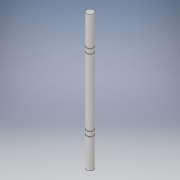
# Autodesk Inventor part: Förderbandwelle_hinten
Saved by Autodesk Inventor 2018 (Build 220112000, 112)
## iProperties
Created: 2017-12-01
Part Number: Förderbandwelle_hinten
Material: Generisch
Document SubType Name: Modeling
Designer: Dominik
Density: 1 g/cm^3
Appearance: Vorgabe
Author: Dominik
Autodesk Inventor part; units mm, degrees
ref_plane "YZ Plane" through (0, 0, 0) normal (1, 0, 0) x (0, 1, 0)
ref_plane "XY Plane" through (0, 0, 0) normal (0, 0, 1) x (1, 0, 0)
sketch "Skizze1" plane through (0, 0, 0) normal (0, 0, 1) x (1, 0, 0)
  circle A0 centre (0, 0) radius 5
  dimension "d0" = 10
  constraints: 1 centre point, 1 coincident
  measures "d0" diameter of A0
extrude "Extrusion1" add sketch "Skizze1" along normal blind 100
sketch "Skizze4" plane through (0, 0, 0) normal (0, 0, -1) x (-1, 0, 0)
  circle A0 centre (0, 0) radius 5
  circle A1 centre (0, 0) radius 5
  dimension "d15" = 10
  constraints: 2 centre point, 2 coincident
  measures "d15" diameter of A0
extrude "Extrusion4" add sketch "Skizze4" along normal blind 50
sketch "Skizze5" plane through (0, 0, 100) normal (0, 0, 1) x (1, 0, 0)
  circle A0 centre (0, 0) radius 5
  constraints: 1 centre point, 1 coincident
extrude "Extrusion5" add sketch "Skizze5" along normal blind 50
ref_plane "Arbeitsebene1" through (0, 5, 0) normal (0, 1, 0) x (-1, 0, 0)
sketch "Skizze6" plane through (0, 5, 0) normal (0, 1, 0) x (-1, 0, 0)
  line L0 (-5, -50) -> (5, -50) projected
  line L1 (0, -50) -> (0, 50)
  line L2 (0, 50) -> (0, 102.85)
  line L3 (0, 50) -> (0, -2.85)
  line L4 (0, -4.35) -> (0, -1.35) construction
  line L5 (1.5, -4.35) -> (1.5, -1.35)
  line L6 (-1.5, -1.35) -> (-1.5, -4.35)
  arc A0 (-1.5, -4.35) -> (1.5, -4.35) centre (0, -4.35) ccw
  arc A1 (1.5, -1.35) -> (-1.5, -1.35) centre (0, -1.35) ccw
  line L7 (0, 101.35) -> (0, 104.35) construction
  line L8 (-1.5, 101.35) -> (-1.5, 104.35)
  line L9 (1.5, 104.35) -> (1.5, 101.35)
  arc A2 (-1.5, 101.35) -> (1.5, 101.35) centre (0, 101.35) ccw
  arc A3 (1.5, 104.35) -> (-1.5, 104.35) centre (0, 104.35) ccw
  point P0 (0, 0)
  dimension "d21" = 100
  dimension "d22" = 52.85
  dimension "d23" = 52.85
  dimension "d27" = 1.5
  dimension "d28" = 6
  dimension "d29" = 1.5
  dimension "d33" = 3
  constraints: 22 end point, 8 point on circle, 8 tangent, 4 centre point, 3 midpoint, 3 point on line, 2 parallel, 2 vertical
  measures "d21" distance of L1.start L1.end
  measures "d22" distance of L1.end L2.end
  measures "d23" distance of L1.end L3.end
  measures "d27" radius of A0
  measures "d29" radius of A3
  measures "d33" distance of L4.start L4.end
extrude "Extrusion6" cut sketch "Skizze6" against normal blind 1.5
ref_plane "Arbeitsebene3" through (0, 5, 105.85) normal (0, 0, 1) x (1, 0, 0)
ref_plane "Arbeitsebene2" through (0, 5, 99.85) normal (0, 0, 1) x (1, 0, 0)
ref_plane "Arbeitsebene5" through (0, 5, -5.85) normal (0, 0, -1) x (-1, 0, 0)
ref_plane "Arbeitsebene4" through (0, 5, 0.15) normal (0, 0, -1) x (-1, 0, 0)
sketch "Skizze7" plane through (0, 5, -5.85) normal (0, 0, -1) x (-1, 0, 0)
  circle A0 centre (0, -5) radius 5
  circle A1 centre (0, -5) radius 3.8
  dimension "d34" = 7.6
  constraints: 2 centre point, 2 coincident
  measures "d34" diameter of A1
extrude "Extrusion7" cut sketch "Skizze7" along normal blind 0.8
sketch "Skizze8" plane through (0, 5, 0.15) normal (0, 0, -1) x (-1, 0, 0)
  circle A0 centre (0, -5) radius 5
  circle A1 centre (0, -5) radius 3.8
  dimension "d37" = 7.6
  constraints: 2 centre point, 2 coincident
  measures "d37" diameter of A1
extrude "Extrusion8" cut sketch "Skizze8" against normal blind 0.8
sketch "Skizze9" plane through (0, 5, 99.85) normal (0, 0, 1) x (1, 0, 0)
  circle A0 centre (0, -5) radius 5
  circle A1 centre (0, -5) radius 3.8
  dimension "d40" = 7.6
  constraints: 2 centre point, 2 coincident
  measures "d40" diameter of A1
extrude "Extrusion9" cut sketch "Skizze9" against normal blind 0.8
sketch "Skizze10" plane through (0, 5, 105.85) normal (0, 0, 1) x (1, 0, 0)
  circle A0 centre (0, -5) radius 5
  circle A1 centre (0, -5) radius 3.8
  constraints: 2 centre point, 2 coincident
extrude "Extrusion10" cut sketch "Skizze10" along normal blind 0.8
